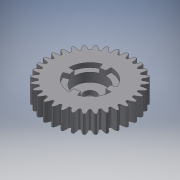
# Autodesk Inventor part: gear 2 clutch
Saved by Autodesk Inventor 2017 (Build 210142000, 142)
## iProperties
Created: 2018-04-17
Part Number: gear 2 clutch
Material: Generic
Document SubType Name: Modeling
Designer: RKL
Density: 1 g/cm^3
Appearance: Default
Author: RKL
Autodesk Inventor part; units mm, degrees
ref_plane "YZ Plane" through (0, 0, 0) normal (1, 0, 0) x (0, 1, 0)
ref_plane "XZ Plane" through (0, 0, 0) normal (0, 1, 0) x (-1, 0, 0)
ref_plane "XY Plane" through (0, 0, 0) normal (0, 0, 1) x (1, 0, 0)
sketch "Sketch1" plane through (0, 0, 0) normal (0, 0, 1) x (1, 0, 0)
  spline S0 degree 3 poles (-3.7304, 46.8517) (-3.5586, 46.5791) (-3.2149, 46.0339) (-2.7481, 45.187) (-2.3226, 44.3184) (-1.9554, 43.4244) (-1.6332, 42.5106) (-1.4979, 41.7141) (-1.2829, 41.1879) (-1.0959, 40.9236) (-0.9158, 40.7608) (-0.7132, 40.6269) (-0.4054, 40.5198) (0, 40.5252) (0.4054, 40.5198) (0.7132, 40.6269) (0.9158, 40.7608) (1.0959, 40.9236) (1.2829, 41.1879) (1.4979, 41.7141) (1.6332, 42.5106) (1.9554, 43.4244) (2.3226, 44.3184) (2.7481, 45.187) (3.2149, 46.0339) (3.5586, 46.5791) (3.7304, 46.8517) knots 0 0 0 0 0.096658 0.193313 0.289967 0.386616 0.483254 0.579874 0.628059 0.652212 0.676357 0.700479 0.724648 0.772816 0.820984 0.845153 0.869275 0.893419 0.917572 0.965758 1.062378 1.159016 1.255665 1.352319 1.448974 1.545632 1.545632 1.545632 1.545632
  circle A0 centre (0, 0) radius 40.523 construction
  circle A1 centre (0, 0) radius 41.3465 construction
  circle A2 centre (0, 0) radius 44 construction
  circle A3 centre (0, 0) radius 47
  point P0 (-3.223, 46.029)
  point P1 (-2.755, 45.1834)
  point P2 (-2.3323, 44.3141)
  point P3 (-1.9629, 43.421)
  point P4 (-1.6598, 42.5034)
  point P5 (-1.4249, 41.5662)
  point P6 (-1.2309, 41.1251)
  point P7 (-1.0893, 40.9295)
  point P8 (-0.912, 40.7656)
  point P9 (-0.7086, 40.6359)
  point P10 (-0.4806, 40.5558)
  point P11 (0, 40.523)
  point P12 (0.4806, 40.5558)
  point P13 (0.7086, 40.6359)
  point P14 (0.912, 40.7656)
  point P15 (1.0893, 40.9295)
  point P16 (1.2309, 41.1251)
  point P17 (1.4249, 41.5662)
  point P18 (1.6598, 42.5034)
  point P19 (1.9629, 43.421)
  point P20 (2.3323, 44.3141)
  point P21 (2.755, 45.1834)
  point P22 (3.223, 46.029)
  constraints: 4 centre point, 2 point on circle, 55 other
extrude "Extrusion1" add sketch "Sketch1" against normal blind 20
extrude "Extrusion2" cut sketch "Sketch1" against normal through all contours A3 S0 picked at (-0.2847, 44.7454)
pattern_circular "Circular Pattern1" count 32 over 360 about axis through (0, 0, 0) along (0, 0, -1) of "Extrusion2"
sketch "Sketch2" plane through (0, 0, 0) normal (0, 0, 1) x (1, 0, 0)
  circle A0 centre (0, 0) radius 6.75
  dimension "d7" = 13.5
  constraints: 1 centre point, 1 coincident
  measures "d7" diameter of A0
extrude "Extrusion3" cut sketch "Sketch2" against normal through all
sketch "Sketch3" plane through (0, 0, 0) normal (0, 0, 1) x (1, 0, 0)
  circle A0 centre (0, 0) radius 17.5
  dimension "d10" = 35
  constraints: 1 centre point, 1 coincident
  measures "d10" diameter of A0
extrude "Extrusion4" cut sketch "Sketch3" against normal blind 15
sketch "Sketch4" plane through (0, 0, 0) normal (0, 0, 1) x (1, 0, 0)
  circle A0 centre (0, 0) radius 17.5 construction
  line L0 (0, 0) -> (0, 17.5) construction
  line L1 (0, 17.5) -> (0, 23.5)
  arc A1 (22.0828, 8.0375) -> (0, 23.5) centre (0, 0) ccw
  arc A2 (16.4446, 5.9854) -> (0, 17.5) centre (0, 0) ccw
  line L2 (22.0828, 8.0375) -> (16.4446, 5.9854)
  dimension "d13" = 6
  dimension "d14" = 70
  constraints: 6 end point, 4 point on circle, 2 centre point, 2 coincident, 1 line through centre, 1 point on line, 1 vertical, 1 vertical alignment, 1 other
  measures "d13" distance of L0.end L1.end
  measures "d14" angle of L2 L1
extrude "Extrusion5" cut sketch "Sketch4" against normal blind 5
pattern_circular "Circular Pattern2" count 4 over 360 about axis through (0, 0, 0) along (0, 0, -1) of "Extrusion5"
equation "\"d0\" = FaceWidth"
equation "\"Module\" = 2.75"
equation "\"PressureAngle\" = 20deg"
equation "\"UnitProfileClearance\" = 0.25"
equation "\"UnitRoundRadius\" = 0.35"
equation "\"HeadDiameter\" = 94"
equation "\"RootDiameter\" = 81.04609"
equation "\"BaseDiameter\" = 82.69295"
equation "\"PitchDiameter\" = 88"
equation "\"FaceWidth\" = 20"
equation "\"HelixAngle\" = 0"
equation "\"UnitCorrection\" = 0.091973"
equation "\"UnitAddendumModification\" = 0.001064"
equation "\"CircularPitch\" = 8.63938"
equation "\"UnitBacklashShift\" = -0.10632"
equation "\"TotalToolShift\" = -0.03945"
equation "\"IsInternal\" = 0"
body "Solid1"
